Autodesk Inventor part; units mm, degrees
(part 2 of 3)
  spline S206 degree 2 poles (86.5499, 10.3817) (86.5499, 12.0564) (88.3061, 14.0423) (89.7214, 14.0423) knots 0 0 0 1 2 2 2
  spline S207 degree 2 poles (89.7214, 14.0423) (90.3587, 14.0423) (91.3442, 13.6718) (91.7073, 13.279) knots 0 0 0 1 2 2 2
  spline S208 degree 2 poles (91.7073, 13.279) (92.0778, 12.8863) (92.4705, 11.7526) (92.4705, 10.93) knots 0 0 0 1 2 2 2
  line L246 (92.4705, 10.93) -> (92.4705, 10.3002)
  line L247 (92.4705, 10.3002) -> (87.7207, 10.3002)
  spline S209 degree 2 poles (87.7207, 10.3002) (87.7207, 9.1072) (88.9211, 7.84) (89.9882, 7.84) knots 0 0 0 1 2 2 2
  spline S210 degree 2 poles (89.9882, 7.84) (90.3661, 7.84) (91.0997, 8.0105) (91.3961, 8.1439) knots 0 0 0 1 2 2 2
  spline S211 degree 2 poles (91.3961, 8.1439) (91.7073, 8.2921) (92.1371, 8.5514) (92.2779, 8.67) knots 0 0 0 1 2 2 2
  line L248 (92.2779, 8.67) -> (92.3446, 8.67)
  line L249 (92.3446, 8.67) -> (92.3446, 7.4103)
  spline S212 degree 2 poles (92.3446, 7.4103) (92.1445, 7.3288) (91.5369, 7.0916) (91.2998, 7.0249) knots 0 0 0 1 2 2 2
  spline S213 degree 2 poles (91.2998, 7.0249) (90.9663, 6.9286) (90.418, 6.8323) (90.003, 6.8323) knots 0 0 0 1 2 2 2
  spline S214 degree 2 poles (91.3442, 11.182) (91.3294, 11.6488) (91.1367, 12.3305) (90.9515, 12.5602) knots 0 0 0 1 2 2 2
  spline S215 degree 2 poles (90.9515, 12.5602) (90.7514, 12.8196) (90.1216, 13.0938) (89.6547, 13.0938) knots 0 0 0 1 2 2 2
  spline S216 degree 2 poles (89.6547, 13.0938) (89.1953, 13.0938) (88.5506, 12.8196) (88.2839, 12.5528) knots 0 0 0 1 2 2 2
  spline S217 degree 2 poles (88.2839, 12.5528) (88.0245, 12.2787) (87.7577, 11.6192) (87.7207, 11.182) knots 0 0 0 1 2 2 2
  line L250 (87.7207, 11.182) -> (91.3442, 11.182)
  line L251 (98.9173, 6.9879) -> (97.7613, 6.9879)
  line L252 (97.7613, 6.9879) -> (97.7613, 7.6844)
  spline S218 degree 2 poles (97.7613, 7.6844) (97.4946, 7.4621) (97.1018, 7.1657) (96.8351, 7.0398) knots 0 0 0 1 2 2 2
  spline S219 degree 2 poles (96.8351, 7.0398) (96.5905, 6.9212) (96.0644, 6.7952) (95.7161, 6.7952) knots 0 0 0 1 2 2 2
  spline S220 degree 2 poles (95.7161, 6.7952) (95.153, 6.7952) (94.2045, 7.2621) (93.871, 7.7141) knots 0 0 0 1 2 2 2
  spline S221 degree 2 poles (93.871, 7.7141) (93.5376, 8.1661) (93.1671, 9.4999) (93.1671, 10.3669) knots 0 0 0 1 2 2 2
  spline S222 degree 2 poles (93.1671, 10.3669) (93.1671, 11.2709) (93.6339, 12.5899) (94.0415, 13.0864) knots 0 0 0 1 2 2 2
  spline S223 degree 2 poles (94.0415, 13.0864) (94.4194, 13.531) (95.479, 14.0423) (96.0644, 14.0423) knots 0 0 0 1 2 2 2
  spline S224 degree 2 poles (96.0644, 14.0423) (96.5757, 14.0423) (97.3389, 13.8125) (97.7613, 13.5754) knots 0 0 0 1 2 2 2
  line L253 (97.7613, 13.5754) -> (97.7613, 16.5394)
  line L254 (97.7613, 16.5394) -> (98.9173, 16.5394)
  line L255 (98.9173, 16.5394) -> (98.9173, 6.9879)
  line L256 (97.7613, 8.6552) -> (97.7613, 12.6195)
  spline S225 degree 2 poles (97.7613, 12.6195) (97.3315, 12.827) (96.6498, 12.9826) (96.2571, 12.9826) knots 0 0 0 1 2 2 2
  spline S226 degree 2 poles (96.2571, 12.9826) (95.3679, 12.9826) (94.3601, 11.6488) (94.3601, 10.3891) knots 0 0 0 1 2 2 2
  spline S227 degree 2 poles (94.3601, 10.3891) (94.3601, 9.1739) (95.1307, 7.8919) (95.9829, 7.8919) knots 0 0 0 1 2 2 2
  spline S228 degree 2 poles (95.9829, 7.8919) (96.4349, 7.8919) (97.3538, 8.3069) (97.7613, 8.6552) knots 0 0 0 1 2 2 2
  line L257 (105.9272, 6.9879) -> (104.7712, 6.9879)
  line L258 (104.7712, 6.9879) -> (104.7712, 7.7437)
  spline S229 degree 2 poles (104.7712, 7.7437) (104.2377, 7.2769) (103.2818, 6.7952) (102.689, 6.7952) knots 0 0 0 1 2 2 2
  spline S230 degree 2 poles (102.689, 6.7952) (102.2444, 6.7952) (101.4515, 7.0916) (101.1625, 7.4103) knots 0 0 0 1 2 2 2
  spline S231 degree 2 poles (101.1625, 7.4103) (100.8661, 7.7289) (100.5401, 8.6996) (100.5401, 9.3962) knots 0 0 0 1 2 2 2
  line L259 (100.5401, 9.3962) -> (100.5401, 13.8496)
  line L260 (100.5401, 13.8496) -> (101.696, 13.8496)
  line L261 (101.696, 13.8496) -> (101.696, 9.9371)
  spline S232 degree 2 poles (101.696, 9.9371) (101.696, 9.3887) (101.7776, 8.67) (101.9184, 8.4032) knots 0 0 0 1 2 2 2
  spline S233 degree 2 poles (101.9184, 8.4032) (102.0591, 8.1365) (102.5408, 7.8919) (102.9928, 7.8919) knots 0 0 0 1 2 2 2
  spline S234 degree 2 poles (102.9928, 7.8919) (103.4152, 7.8919) (104.3711, 8.3736) (104.7712, 8.7218) knots 0 0 0 1 2 2 2
  line L262 (104.7712, 8.7218) -> (104.7712, 13.8496)
  line L263 (104.7712, 13.8496) -> (105.9272, 13.8496)
  line L264 (105.9272, 13.8496) -> (105.9272, 6.9879)
  line L265 (143.2657, 28.3705) -> (142.0505, 28.3705)
  line L266 (142.0505, 28.3705) -> (142.0505, 36.2474)
  line L267 (142.0505, 36.2474) -> (139.6645, 30.8899)
  line L268 (139.6645, 30.8899) -> (138.9235, 30.8899)
  line L269 (138.9235, 30.8899) -> (136.5597, 36.2474)
  line L270 (136.5597, 36.2474) -> (136.5597, 28.3705)
  line L271 (136.5597, 28.3705) -> (135.4259, 28.3705)
  line L272 (135.4259, 28.3705) -> (135.4259, 37.5145)
  line L273 (135.4259, 37.5145) -> (137.0858, 37.5145)
  line L274 (137.0858, 37.5145) -> (139.3681, 32.4238)
  line L275 (139.3681, 32.4238) -> (141.5763, 37.5145)
  line L276 (141.5763, 37.5145) -> (143.2657, 37.5145)
  line L277 (143.2657, 37.5145) -> (143.2657, 28.3705)
  spline S235 degree 2 poles (148.312, 28.1778) (147.5043, 28.1778) (146.3039, 28.6002) (145.8815, 29.0226) knots 0 0 0 1 2 2 2
  spline S236 degree 2 poles (145.8815, 29.0226) (145.3998, 29.4968) (145.0071, 30.8306) (145.0071, 31.8088) knots 0 0 0 1 2 2 2
  line L278 (145.0071, 31.8088) -> (145.0071, 37.5145)
  line L279 (145.0071, 37.5145) -> (146.2224, 37.5145)
  line L280 (146.2224, 37.5145) -> (146.2224, 31.8088)
  spline S237 degree 2 poles (146.2224, 31.8088) (146.2224, 31.1715) (146.3854, 30.3119) (146.6151, 29.9637) knots 0 0 0 1 2 2 2
  spline S238 degree 2 poles (146.6151, 29.9637) (146.8596, 29.5932) (147.7044, 29.2152) (148.312, 29.2152) knots 0 0 0 1 2 2 2
  spline S239 degree 2 poles (148.312, 29.2152) (148.8826, 29.2152) (149.7718, 29.5932) (150.0163, 29.9637) knots 0 0 0 1 2 2 2
  spline S240 degree 2 poles (150.0163, 29.9637) (150.246, 30.3119) (150.409, 31.1641) (150.409, 31.7791) knots 0 0 0 1 2 2 2
  line L281 (150.409, 31.7791) -> (150.409, 37.5145)
  line L282 (150.409, 37.5145) -> (151.6243, 37.5145)
  line L283 (151.6243, 37.5145) -> (151.6243, 31.8088)
  spline S241 degree 2 poles (151.6243, 31.8088) (151.6243, 30.8529) (151.239, 29.4894) (150.7499, 29.0226) knots 0 0 0 1 2 2 2
  spline S242 degree 2 poles (150.7499, 29.0226) (150.3127, 28.5928) (149.1567, 28.1778) (148.312, 28.1778) knots 0 0 0 1 2 2 2
  spline S243 degree 2 poles (155.9147, 28.2075) (154.9218, 28.2075) (153.5287, 28.6224) (152.9136, 28.9188) knots 0 0 0 1 2 2 2
  line L284 (152.9136, 28.9188) -> (152.9136, 30.4453)
  line L285 (152.9136, 30.4453) -> (153.0026, 30.4453)
  spline S244 degree 2 poles (153.0026, 30.4453) (153.6028, 29.8821) (155.1218, 29.2597) (155.8258, 29.2597) knots 0 0 0 1 2 2 2
  spline S245 degree 2 poles (155.8258, 29.2597) (156.8335, 29.2597) (157.8635, 30.097) (157.8635, 30.7862) knots 0 0 0 1 2 2 2
  spline S246 degree 2 poles (157.8635, 30.7862) (157.8635, 31.3345) (157.3226, 32.0162) (156.7372, 32.1867) knots 0 0 0 1 2 2 2
  spline S247 degree 2 poles (156.7372, 32.1867) (156.3148, 32.3052) (155.6109, 32.4683) (155.0848, 32.6016) knots 0 0 0 1 2 2 2
  spline S248 degree 2 poles (155.0848, 32.6016) (154.6105, 32.7276) (153.8621, 33.1055) (153.5731, 33.4093) knots 0 0 0 1 2 2 2
  spline S249 degree 2 poles (153.5731, 33.4093) (153.2915, 33.7131) (152.9803, 34.5282) (152.9803, 35.0618) knots 0 0 0 1 2 2 2
  spline S250 degree 2 poles (152.9803, 35.0618) (152.9803, 36.1733) (154.7143, 37.6775) (156.0555, 37.6775) knots 0 0 0 1 2 2 2
  spline S251 degree 2 poles (156.0555, 37.6775) (156.8261, 37.6775) (158.1896, 37.3737) (158.775, 37.0847) knots 0 0 0 1 2 2 2
  line L286 (158.775, 37.0847) -> (158.775, 35.6323)
  line L287 (158.775, 35.6323) -> (158.6861, 35.6323)
  spline S252 degree 2 poles (158.6861, 35.6323) (158.2489, 36.0325) (156.8854, 36.6253) (156.137, 36.6253) knots 0 0 0 1 2 2 2
  spline S253 degree 2 poles (156.137, 36.6253) (155.2923, 36.6253) (154.2474, 35.8324) (154.2474, 35.1877) knots 0 0 0 1 2 2 2
  spline S254 degree 2 poles (154.2474, 35.1877) (154.2474, 34.6098) (154.8625, 33.9206) (155.4405, 33.765) knots 0 0 0 1 2 2 2
  spline S255 degree 2 poles (155.4405, 33.765) (155.8258, 33.6613) (156.9447, 33.3945) (157.3152, 33.2834) knots 0 0 0 1 2 2 2
  spline S256 degree 2 poles (157.3152, 33.2834) (158.2563, 32.9944) (159.1307, 31.831) (159.1307, 30.9788) knots 0 0 0 1 2 2 2
  spline S257 degree 2 poles (159.1307, 30.9788) (159.1307, 30.4379) (158.6935, 29.4005) (158.3007, 29.0374) knots 0 0 0 1 2 2 2
  spline S258 degree 2 poles (158.3007, 29.0374) (157.8635, 28.6373) (156.752, 28.2075) (155.9147, 28.2075) knots 0 0 0 1 2 2 2
  line L288 (169.2157, 28.3705) -> (164.7549, 28.3705)
  line L289 (164.7549, 28.3705) -> (164.7549, 29.3042)
  line L290 (164.7549, 29.3042) -> (166.4147, 29.3042)
  line L291 (166.4147, 29.3042) -> (166.4147, 35.4323)
  line L292 (166.4147, 35.4323) -> (164.7549, 35.4323)
  line L293 (164.7549, 35.4323) -> (164.7549, 36.2696)
  spline S259 degree 2 poles (164.7549, 36.2696) (165.696, 36.2696) (166.5852, 36.8031) (166.6444, 37.5441) knots 0 0 0 1 2 2 2
  line L294 (166.6444, 37.5441) -> (167.5929, 37.5441)
  line L295 (167.5929, 37.5441) -> (167.5929, 29.3042)
  line L296 (167.5929, 29.3042) -> (169.2157, 29.3042)
  line L297 (169.2157, 29.3042) -> (169.2157, 28.3705)
  line L298 (170.1716, 28.3705) -> (173.2542, 37.5145)
  line L299 (173.2542, 37.5145) -> (174.751, 37.5145)
  line L300 (174.751, 37.5145) -> (177.8336, 28.3705)
  line L301 (177.8336, 28.3705) -> (176.5517, 28.3705)
  line L302 (176.5517, 28.3705) -> (175.7218, 30.927)
  line L303 (175.7218, 30.927) -> (172.2316, 30.927)
  line L304 (172.2316, 30.927) -> (171.4017, 28.3705)
  line L305 (171.4017, 28.3705) -> (170.1716, 28.3705)
  line L306 (175.3883, 31.9644) -> (173.973, 36.2696)
  line L307 (173.973, 36.2696) -> (172.5651, 31.9644)
  line L308 (172.5651, 31.9644) -> (175.3883, 31.9644)
  spline S260 degree 2 poles (121.6729, 13.1521) (120.6799, 13.1521) (119.2868, 13.5671) (118.6718, 13.8635) knots 0 0 0 1 2 2 2
  line L309 (118.6718, 13.8635) -> (118.6718, 15.39)
  line L310 (118.6718, 15.39) -> (118.7607, 15.39)
  spline S261 degree 2 poles (118.7607, 15.39) (119.3609, 14.8268) (120.88, 14.2043) (121.5839, 14.2043) knots 0 0 0 1 2 2 2
  spline S262 degree 2 poles (121.5839, 14.2043) (122.5917, 14.2043) (123.6217, 15.0417) (123.6217, 15.7308) knots 0 0 0 1 2 2 2
  spline S263 degree 2 poles (123.6217, 15.7308) (123.6217, 16.2792) (123.0808, 16.9609) (122.4954, 17.1313) knots 0 0 0 1 2 2 2
  spline S264 degree 2 poles (122.4954, 17.1313) (122.073, 17.2499) (121.3691, 17.4129) (120.8429, 17.5463) knots 0 0 0 1 2 2 2
  spline S265 degree 2 poles (120.8429, 17.5463) (120.3687, 17.6723) (119.6203, 18.0502) (119.3313, 18.354) knots 0 0 0 1 2 2 2
  spline S266 degree 2 poles (119.3313, 18.354) (119.0497, 18.6578) (118.7385, 19.4729) (118.7385, 20.0064) knots 0 0 0 1 2 2 2
  spline S267 degree 2 poles (118.7385, 20.0064) (118.7385, 21.1179) (120.4724, 22.6222) (121.8137, 22.6222) knots 0 0 0 1 2 2 2
  spline S268 degree 2 poles (121.8137, 22.6222) (122.5843, 22.6222) (123.9478, 22.3184) (124.5331, 22.0294) knots 0 0 0 1 2 2 2
  line L311 (124.5331, 22.0294) -> (124.5331, 20.577)
  line L312 (124.5331, 20.577) -> (124.4442, 20.577)
  spline S269 degree 2 poles (124.4442, 20.577) (124.007, 20.9771) (122.6436, 21.5699) (121.8952, 21.5699) knots 0 0 0 1 2 2 2
  spline S270 degree 2 poles (121.8952, 21.5699) (121.0504, 21.5699) (120.0056, 20.7771) (120.0056, 20.1324) knots 0 0 0 1 2 2 2
  spline S271 degree 2 poles (120.0056, 20.1324) (120.0056, 19.5544) (120.6206, 18.8653) (121.1986, 18.7097) knots 0 0 0 1 2 2 2
  spline S272 degree 2 poles (121.1986, 18.7097) (121.5839, 18.6059) (122.7029, 18.3392) (123.0734, 18.228) knots 0 0 0 1 2 2 2
  spline S273 degree 2 poles (123.0734, 18.228) (124.0144, 17.939) (124.8888, 16.7756) (124.8888, 15.9235) knots 0 0 0 1 2 2 2
  spline S274 degree 2 poles (124.8888, 15.9235) (124.8888, 15.3825) (124.4516, 14.3451) (124.0589, 13.982) knots 0 0 0 1 2 2 2
  spline S275 degree 2 poles (124.0589, 13.982) (123.6217, 13.5819) (122.5102, 13.1521) (121.6729, 13.1521) knots 0 0 0 1 2 2 2
  line L313 (126.1263, 13.3151) -> (126.1263, 22.4591)
  line L314 (126.1263, 22.4591) -> (131.8469, 22.4591)
  line L315 (131.8469, 22.4591) -> (131.8469, 21.3773)
  line L316 (131.8469, 21.3773) -> (127.3416, 21.3773)
  line L317 (127.3416, 21.3773) -> (127.3416, 18.8727)
  line L318 (127.3416, 18.8727) -> (131.5431, 18.8727)
  line L319 (131.5431, 18.8727) -> (131.5431, 17.7908)
  line L320 (131.5431, 17.7908) -> (127.3416, 17.7908)
  line L321 (127.3416, 17.7908) -> (127.3416, 14.397)
  line L322 (127.3416, 14.397) -> (131.8469, 14.397)
  line L323 (131.8469, 14.397) -> (131.8469, 13.3151)
  line L324 (131.8469, 13.3151) -> (126.1263, 13.3151)
  spline S276 degree 2 poles (136.7523, 13.1521) (135.8631, 13.1521) (134.3589, 13.7523) (133.8105, 14.3525) knots 0 0 0 1 2 2 2
  spline S277 degree 2 poles (133.8105, 14.3525) (133.2622, 14.9454) (132.662, 16.7238) (132.662, 17.8797) knots 0 0 0 1 2 2 2
  spline S278 degree 2 poles (132.662, 17.8797) (132.662, 19.0283) (133.2474, 20.7326) (133.8031, 21.3625) knots 0 0 0 1 2 2 2
  spline S279 degree 2 poles (133.8031, 21.3625) (134.3515, 21.9775) (135.8483, 22.6222) (136.7745, 22.6222) knots 0 0 0 1 2 2 2
  spline S280 degree 2 poles (136.7745, 22.6222) (137.234, 22.6222) (138.0417, 22.4888) (138.3825, 22.385) knots 0 0 0 1 2 2 2
  spline S281 degree 2 poles (138.3825, 22.385) (138.6789, 22.2887) (139.294, 22.0145) (139.5978, 21.8515) knots 0 0 0 1 2 2 2
  line L325 (139.5978, 21.8515) -> (139.5978, 20.3843)
  line L326 (139.5978, 20.3843) -> (139.5014, 20.3843)
  spline S282 degree 2 poles (139.5014, 20.3843) (139.3384, 20.5325) (138.8345, 20.9475) (138.4714, 21.1476) knots 0 0 0 1 2 2 2
  spline S283 degree 2 poles (138.4714, 21.1476) (138.1232, 21.3402) (137.3007, 21.5848) (136.7671, 21.5848) knots 0 0 0 1 2 2 2
  spline S284 degree 2 poles (136.7671, 21.5848) (136.1817, 21.5848) (135.1369, 21.1031) (134.7442, 20.6437) knots 0 0 0 1 2 2 2
  spline S285 degree 2 poles (134.7442, 20.6437) (134.3589, 20.1768) (133.9291, 18.7615) (133.9291, 17.8797) knots 0 0 0 1 2 2 2
  spline S286 degree 2 poles (133.9291, 17.8797) (133.9291, 16.9387) (134.3811, 15.5826) (134.7738, 15.1158) knots 0 0 0 1 2 2 2
  spline S287 degree 2 poles (134.7738, 15.1158) (135.1592, 14.6638) (136.1892, 14.2043) (136.7671, 14.2043) knots 0 0 0 1 2 2 2
  spline S288 degree 2 poles (136.7671, 14.2043) (137.2933, 14.2043) (138.1899, 14.4637) (138.5381, 14.6564) knots 0 0 0 1 2 2 2
  spline S289 degree 2 poles (138.5381, 14.6564) (138.8716, 14.849) (139.3681, 15.2492) (139.5089, 15.39) knots 0 0 0 1 2 2 2
  line L327 (139.5089, 15.39) -> (139.5978, 15.39)
  line L328 (139.5978, 15.39) -> (139.5978, 13.9376)
  spline S290 degree 2 poles (139.5978, 13.9376) (139.294, 13.7968) (138.7604, 13.5374) (138.3825, 13.4189) knots 0 0 0 1 2 2 2
  spline S291 degree 2 poles (138.3825, 13.4189) (137.9824, 13.2855) (137.3007, 13.1521) (136.7523, 13.1521) knots 0 0 0 1 2 2 2
  line L329 (142.8656, 13.3151) -> (142.8656, 21.3773)
  line L330 (142.8656, 21.3773) -> (139.7978, 21.3773)
  line L331 (139.7978, 21.3773) -> (139.7978, 22.4591)
  line L332 (139.7978, 22.4591) -> (147.1486, 22.4591)
  line L333 (147.1486, 22.4591) -> (147.1486, 21.3773)
  line L334 (147.1486, 21.3773) -> (144.0809, 21.3773)
  line L335 (144.0809, 21.3773) -> (144.0809, 13.3151)
  line L336 (144.0809, 13.3151) -> (142.8656, 13.3151)
  line L337 (151.2612, 13.3151) -> (147.7192, 13.3151)
  line L338 (147.7192, 13.3151) -> (147.7192, 14.2488)
  line L339 (147.7192, 14.2488) -> (148.8826, 14.2488)
  line L340 (148.8826, 14.2488) -> (148.8826, 21.5255)
  line L341 (148.8826, 21.5255) -> (147.7192, 21.5255)
  line L342 (147.7192, 21.5255) -> (147.7192, 22.4591)
  line L343 (147.7192, 22.4591) -> (151.2612, 22.4591)
  line L344 (151.2612, 22.4591) -> (151.2612, 21.5255)
  line L345 (151.2612, 21.5255) -> (150.0978, 21.5255)
  line L346 (150.0978, 21.5255) -> (150.0978, 14.2488)
  line L347 (150.0978, 14.2488) -> (151.2612, 14.2488)
  line L348 (151.2612, 14.2488) -> (151.2612, 13.3151)
  spline S292 degree 2 poles (159.2344, 21.4143) (159.7531, 20.8067) (160.3311, 19.0283) (160.3311, 17.8871) knots 0 0 0 1 2 2 2
  spline S293 degree 2 poles (160.3311, 17.8871) (160.3311, 16.7756) (159.7679, 14.975) (159.2344, 14.3674) knots 0 0 0 1 2 2 2
  spline S294 degree 2 poles (159.2344, 14.3674) (158.6712, 13.7301) (157.1818, 13.1225) (156.2852, 13.1225) knots 0 0 0 1 2 2 2
  spline S295 degree 2 poles (156.2852, 13.1225) (155.3589, 13.1225) (153.8769, 13.7523) (153.336, 14.3674) knots 0 0 0 1 2 2 2
  spline S296 degree 2 poles (153.336, 14.3674) (152.8099, 14.975) (152.2467, 16.7608) (152.2467, 17.8871) knots 0 0 0 1 2 2 2
  spline S297 degree 2 poles (152.2467, 17.8871) (152.2467, 19.0357) (152.8173, 20.7845) (153.3434, 21.4143) knots 0 0 0 1 2 2 2
  spline S298 degree 2 poles (153.3434, 21.4143) (153.8769, 22.0219) (155.3664, 22.6518) (156.2852, 22.6518) knots 0 0 0 1 2 2 2
  spline S299 degree 2 poles (156.2852, 22.6518) (157.2189, 22.6518) (158.7157, 21.9997) (159.2344, 21.4143) knots 0 0 0 1 2 2 2
  spline S300 degree 2 poles (159.064, 17.8871) (159.064, 18.7912) (158.6712, 20.1917) (158.3156, 20.6511) knots 0 0 0 1 2 2 2
  spline S301 degree 2 poles (158.3156, 20.6511) (157.9525, 21.1253) (156.9299, 21.5996) (156.2926, 21.5996) knots 0 0 0 1 2 2 2
  spline S302 degree 2 poles (156.2926, 21.5996) (155.6331, 21.5996) (154.6402, 21.1402) (154.2623, 20.6511) knots 0 0 0 1 2 2 2
  spline S303 degree 2 poles (154.2623, 20.6511) (153.8992, 20.1843) (153.5138, 18.7763) (153.5138, 17.8871) knots 0 0 0 1 2 2 2
  spline S304 degree 2 poles (153.5138, 17.8871) (153.5138, 16.0865) (155.0255, 14.1747) (156.2926, 14.1747) knots 0 0 0 1 2 2 2
  spline S305 degree 2 poles (156.2926, 14.1747) (157.5597, 14.1747) (159.064, 16.0865) (159.064, 17.8871) knots 0 0 0 1 2 2 2
  line L349 (168.208, 13.3151) -> (166.8445, 13.3151)
  line L350 (166.8445, 13.3151) -> (162.7986, 21.1994)
  line L351 (162.7986, 21.1994) -> (162.7986, 13.3151)
  line L352 (162.7986, 13.3151) -> (161.6649, 13.3151)
  line L353 (161.6649, 13.3151) -> (161.6649, 22.4591)
  line L354 (161.6649, 22.4591) -> (163.3914, 22.4591)
  line L355 (163.3914, 22.4591) -> (167.0742, 15.2195)
  line L356 (167.0742, 15.2195) -> (167.0742, 22.4591)
  line L357 (167.0742, 22.4591) -> (168.208, 22.4591)
  line L358 (168.208, 22.4591) -> (168.208, 13.3151)
  spline S306 degree 2 poles (180.19, 16.1236) (180.19, 15.4418) (179.6713, 14.397) (179.2415, 14.0561) knots 0 0 0 1 2 2 2
  spline S307 degree 2 poles (179.2415, 14.0561) (178.7228, 13.656) (177.5446, 13.3151) (176.611, 13.3151) knots 0 0 0 1 2 2 2
  line L359 (176.611, 13.3151) -> (173.9878, 13.3151)
  line L360 (173.9878, 13.3151) -> (173.9878, 22.4591)
  line L361 (173.9878, 22.4591) -> (176.4109, 22.4591)
  spline S308 degree 2 poles (176.4109, 22.4591) (177.389, 22.4591) (178.3671, 22.3332) (178.8118, 22.0886) knots 0 0 0 1 2 2 2
  spline S309 degree 2 poles (178.8118, 22.0886) (179.3082, 21.8293) (179.7602, 20.9771) (179.7602, 20.3991) knots 0 0 0 1 2 2 2
  spline S310 degree 2 poles (179.7602, 20.3991) (179.7602, 19.7545) (179.0785, 18.7319) (178.4783, 18.4429) knots 0 0 0 1 2 2 2
  line L362 (178.4783, 18.4429) -> (178.4783, 18.3984)
  spline S311 degree 2 poles (178.4783, 18.3984) (179.2934, 18.1761) (180.19, 16.9979) (180.19, 16.1236) knots 0 0 0 1 2 2 2
  spline S312 degree 2 poles (178.9229, 16.0717) (178.9229, 16.5904) (178.6265, 17.2573) (178.1819, 17.4944) knots 0 0 0 1 2 2 2
  spline S313 degree 2 poles (178.1819, 17.4944) (177.8929, 17.6426) (177.2112, 17.7315) (176.5813, 17.7315) knots 0 0 0 1 2 2 2
  line L363 (176.5813, 17.7315) -> (175.2031, 17.7315)
  line L364 (175.2031, 17.7315) -> (175.2031, 14.3525)
  line L365 (175.2031, 14.3525) -> (176.1886, 14.3525)
  spline S314 degree 2 poles (176.1886, 14.3525) (176.9889, 14.3525) (177.9077, 14.5008) (178.2634, 14.7379) knots 0 0 0 1 2 2 2
  spline S315 degree 2 poles (178.2634, 14.7379) (178.6043, 14.9824) (178.9229, 15.59) (178.9229, 16.0717) knots 0 0 0 1 2 2 2
  spline S316 degree 2 poles (178.4931, 20.2287) (178.4931, 20.5548) (178.2708, 21.0438) (178.0263, 21.1846) knots 0 0 0 1 2 2 2
  spline S317 degree 2 poles (178.0263, 21.1846) (177.7299, 21.3476) (177.0111, 21.4217) (176.3664, 21.4217) knots 0 0 0 1 2 2 2
  line L366 (176.3664, 21.4217) -> (175.2031, 21.4217)
  line L367 (175.2031, 21.4217) -> (175.2031, 18.7467)
  line L368 (175.2031, 18.7467) -> (176.5813, 18.7467)
  spline S318 degree 2 poles (176.5813, 18.7467) (177.1519, 18.7467) (177.6928, 18.8653) (177.9818, 19.0505) knots 0 0 0 1 2 2 2
  spline S319 degree 2 poles (177.9818, 19.0505) (178.2634, 19.2284) (178.4931, 19.7989) (178.4931, 20.2287) knots 0 0 0 1 2 2 2
  spline S320 degree 2 poles (186.8294, 17.8871) (186.8294, 15.427) (185.3993, 13.1225) (183.9099, 13.1225) knots 0 0 0 1 2 2 2
  spline S321 degree 2 poles (183.9099, 13.1225) (182.3982, 13.1225) (180.9829, 15.4715) (180.9829, 17.8797) knots 0 0 0 1 2 2 2
  spline S322 degree 2 poles (180.9829, 17.8797) (180.9829, 20.3547) (182.413, 22.6444) (183.9099, 22.6444) knots 0 0 0 1 2 2 2
  spline S323 degree 2 poles (183.9099, 22.6444) (185.4141, 22.6444) (186.8294, 20.2732) (186.8294, 17.8871) knots 0 0 0 1 2 2 2
  spline S324 degree 2 poles (185.2585, 15.101) (185.4363, 15.553) (185.5845, 16.9461) (185.5845, 17.8871) knots 0 0 0 1 2 2 2
  spline S325 degree 2 poles (185.5845, 17.8871) (185.5845, 18.8282) (185.4363, 20.2139) (185.2511, 20.6807) knots 0 0 0 1 2 2 2
  spline S326 degree 2 poles (185.2511, 20.6807) (185.0658, 21.1476) (184.4212, 21.6292) (183.9099, 21.6292) knots 0 0 0 1 2 2 2
  spline S327 degree 2 poles (183.9099, 21.6292) (183.3986, 21.6292) (182.7391, 21.1476) (182.5464, 20.6659) knots 0 0 0 1 2 2 2
  spline S328 degree 2 poles (182.5464, 20.6659) (182.3612, 20.1991) (182.2278, 18.7763) (182.2278, 17.8797) knots 0 0 0 1 2 2 2
  spline S329 degree 2 poles (182.2278, 17.8797) (182.2278, 16.9164) (182.3463, 15.6271) (182.539, 15.1232) knots 0 0 0 1 2 2 2
  spline S330 degree 2 poles (182.539, 15.1232) (182.7168, 14.649) (183.3763, 14.1377) (183.9099, 14.1377) knots 0 0 0 1 2 2 2
  spline S331 degree 2 poles (183.9099, 14.1377) (184.4137, 14.1377) (185.0732, 14.6193) (185.2585, 15.101) knots 0 0 0 1 2 2 2
  spline S332 degree 2 poles (190.4678, 21.5922) (190.1343, 21.5922) (189.4748, 21.4291) (189.1562, 21.3032) knots 0 0 0 1 2 2 2
  spline S333 degree 2 poles (189.1562, 21.3032) (188.8598, 21.1772) (188.4226, 20.9104) (188.2522, 20.7919) knots 0 0 0 1 2 2 2
  line L369 (188.2522, 20.7919) -> (188.1781, 20.7919)
  line L370 (188.1781, 20.7919) -> (188.1781, 22.0886)
  spline S334 degree 2 poles (188.1781, 22.0886) (188.5782, 22.3035) (189.9491, 22.6518) (190.5641, 22.6518) knots 0 0 0 1 2 2 2
  spline S335 degree 2 poles (190.5641, 22.6518) (191.1865, 22.6518) (192.1128, 22.3999) (192.4907, 22.1331) knots 0 0 0 1 2 2 2
  spline S336 degree 2 poles (192.4907, 22.1331) (192.8908, 21.8441) (193.3058, 21.0068) (193.3058, 20.4436) knots 0 0 0 1 2 2 2
  spline S337 degree 2 poles (193.3058, 20.4436) (193.3058, 19.6878) (192.3129, 18.5466) (191.6163, 18.3984) knots 0 0 0 1 2 2 2
  line L371 (191.6163, 18.3984) -> (191.6163, 18.3095)
  spline S338 degree 2 poles (191.6163, 18.3095) (191.9053, 18.2502) (192.5648, 17.9835) (192.8464, 17.7167) knots 0 0 0 1 2 2 2
  spline S339 degree 2 poles (192.8464, 17.7167) (193.128, 17.4574) (193.4836, 16.6274) (193.4836, 16.0272) knots 0 0 0 1 2 2 2
  spline S340 degree 2 poles (193.4836, 16.0272) (193.4836, 15.4122) (193.0613, 14.3674) (192.676, 13.9672) knots 0 0 0 1 2 2 2
  spline S341 degree 2 poles (192.676, 13.9672) (192.2758, 13.5523) (191.1421, 13.1225) (190.4233, 13.1225) knots 0 0 0 1 2 2 2
  spline S342 degree 2 poles (190.4233, 13.1225) (189.7342, 13.1225) (188.3855, 13.4559) (187.9261, 13.6856) knots 0 0 0 1 2 2 2
  line L372 (187.9261, 13.6856) -> (187.9261, 14.9824)
  line L373 (187.9261, 14.9824) -> (188.015, 14.9824)
  spline S343 degree 2 poles (188.015, 14.9824) (188.4004, 14.7008) (189.7045, 14.1821) (190.3492, 14.1821) knots 0 0 0 1 2 2 2
  spline S344 degree 2 poles (190.3492, 14.1821) (190.7271, 14.1821) (191.4829, 14.4192) (191.7349, 14.6934) knots 0 0 0 1 2 2 2
  spline S345 degree 2 poles (191.7349, 14.6934) (191.9794, 14.9676) (192.2388, 15.6197) (192.2388, 16.1161) knots 0 0 0 1 2 2 2
  spline S346 degree 2 poles (192.2388, 16.1161) (192.2388, 16.6126) (191.9498, 17.2573) (191.6904, 17.4425) knots 0 0 0 1 2 2 2
  spline S347 degree 2 poles (191.6904, 17.4425) (191.4311, 17.6278) (190.7271, 17.7686) (190.3121, 17.7686) knots 0 0 0 1 2 2 2
  line L374 (190.3121, 17.7686) -> (189.7934, 17.7686)
  line L375 (189.7934, 17.7686) -> (189.7934, 18.7838)
  line L376 (189.7934, 18.7838) -> (190.201, 18.7838)
  spline S348 degree 2 poles (190.201, 18.7838) (191.0235, 18.7838) (192.0609, 19.5692) (192.0609, 20.3176) knots 0 0 0 1 2 2 2
  spline S349 degree 2 poles (192.0609, 20.3176) (192.0609, 20.6659) (191.7942, 21.1624) (191.5793, 21.3106) knots 0 0 0 1 2 2 2
  spline S350 degree 2 poles (191.5793, 21.3106) (191.3496, 21.4662) (190.7864, 21.5922) (190.4678, 21.5922) knots 0 0 0 1 2 2 2
  dimension "d10" = 203.2
  dimension "d11" = 50.8
  dimension "d12" = 80.6634
  dimension "d13" = 24.7194
  dimension "d14" = 102.5205
  dimension "d15" = 45.5358
  dimension "d16" = 2.6321
  dimension "d17" = 13.0403
  dimension "d18" = 6.672
  dimension "d19" = 6.672
  constraints: 4 other
  measures "d10" distance of L0.end L1.end
  measures "d11" distance of L1.end L2.end
  measures "d12" distance of L8.start L8.end
  measures "d13" distance of L10.end L8.start
  measures "d14" distance of L4.start L4.end
  measures "d15" distance of L6.end L4.start
  measures "d16" distance between parallel lines of L1 L4
  measures "d17" distance between parallel lines of L1 L8
  measures "d18" distance between parallel lines of L2 L7
  measures "d19" distance between parallel lines of L5 L11
extrude "Extrusion3" cut sketch "Sketch3" against normal blind 5.08 contours S0 S1 L12 L13 S2 S3 S4 L14 L15 L16 L17 L18 | S5 S6 L19 L20 L21 S7 S8 S9 S10 L22 L23 L24 S11 S12 | S13 L25 L26 S14 S15 S16 S17 S18 S19 S20 S21 L27 L28 S22 S23 S24 S25 S26 S27 S28 | L29 L30 L31 L32 L33 L34 L35 L36 | L37 L38 L39 L40 L41 L42 L43 L44 L45 L46 L47 L48 | L49 L50 L51 L52 L53 L54 L55 L56 L57 L58 | L59 L60 L61 L62 L63 L64 L65 L66 | L70 L71 L72 L73 L74 L75 | L76 L77 L78 L79 L80 L81 | L82 L83 L84 L85 L86 L87 L88 L89 L90 L91 L92 L93 | L94 L95 L96 L97 L98 L99 L100 L101 L102 L103 | L104 L105 L106 L107 L108 L109 L110 L111 | L115 L116 L117 L118 L119 L120 S29 L121 L122 L123 L124 | L125 L126 L127 L128 L129 L130 L131 L132 L133 L134 L135 | S30 S31 S32 L139 L140 S33 S34 S35 S36 S37 S38 S39 L141 L142 L143 L144 L145 S40 S41 S42 | S43 S44 S45 S46 S47 S48 S49 L146 L147 S50 S51 S52 S53 S54 | S62 S63 S64 S65 S66 S67 S68 L148 L149 S69 S70 S71 S72 S73 | S81 S82 S83 S84 | L150 L151 L152 L153 L154 L155 L156 | L157 L158 L159 L160 L161 L162 S93 L163 L164 L165 L166 | S94 S95 L167 L168 S96 S97 S98 L169 L170 L171 L172 L173 | L174 L175 L176 L177 | S99 S100 L178 L179 L180 L181 L182 S101 S102 | S107 S108 S109 S110 S111 S112 L184 S113 S114 S115 L185 L186 S116 S117 S118 L187 L188 L189 | L191 L192 L193 L194 | L195 L196 L197 L198 | S123 S124 S125 S126 L199 L200 S127 S128 S129 L201 L202 S130 S131 | L204 L205 S136 S137 S138 L206 L207 L208 L209 L210 S139 S140 L211 | S141 L212 L213 S142 S143 S144 S145 L214 L215 L216 L217 S146 S147 S148 S149 S150 L218 S151 S152 S153 S154 | L220 L221 S159 S160 S161 L222 L223 L224 S162 S163 S164 L225 L226 L227 | S165 S166 S167 S168 S169 L228 L229 S170 S171 S172 S173 S174 L230 L231 S175 S176 | S177 L232 L233 S178 S179 S180 S181 S182 S183 S184 S185 S186 L234 L235 S187 S188 S189 S190 S191 S192 S193 | L236 L237 S194 S195 S196 S197 S198 S199 S200 L238 L239 L240 | L242 L243 L244 L245 | S205 S206 S207 S208 L246 L247 S209 S210 S211 L248 L249 S212 S213 | L251 L252 S218 S219 S220 S221 S222 S223 S224 L253 L254 L255 | L257 L258 S229 S230 S231 L259 L260 L261 S232 S233 S234 L262 L263 L264 | L265 L266 L267 L268 L269 L270 L271 L272 L273 L274 L275 L276 L277 | S235 S236 L278 L279 L280 S237 S238 S239 S240 L281 L282 L283 S241 S242 | S243 L284 L285 S244 S245 S246 S247 S248 S249 S250 S251 L286 L287 S252 S253 S254 S255 S256 S257 S258 | L288 L289 L290 L291 L292 L293 S259 L294 L295 L296 L297 | L298 L299 L300 L301 L302 L303 L304 L305 | S260 L309 L310 S261 S262 S263 S264 S265 S266 S267 S268 L311 L312 S269 S270 S271 S272 S273 S274 S275 | L313 L314 L315 L316 L317 L318 L319 L320 L321 L322 L323 L324 | S276 S277 S278 S279 S280 S281 L325 L326 S282 S283 S284 S285 S286 S287 S288 S289 L327 L328 S290 S291 | L329 L330 L331 L332 L333 L334 L335 L336 | L337 L338 L339 L340 L341 L342 L343 L344 L345 L346 L347 L348 | S292 S293 S294 S295 S296 S297 S298 S299 | L349 L350 L351 L352 L353 L354 L355 L356 L357 L358 | S306 S307 L359 L360 L361 S308 S309 S310 L362 S311 | S320 S321 S322 S323 | S332 S333 L369 L370 S334 S335 S336 S337 L371 S338 S339 S340 S341 S342 L372 L373 S343 S344 S345 S346 S347 L374 L375 L376 S348 S349 S350
sketch "Sketch4" plane through (203.2, 0, 50.8) normal (1, 0, 0) x (0, 0, -1)
  line L0 (0, 0) -> (50.8, 0) projected
  line L1 (0, 0) -> (0, -25.4) projected
  line L2 (50.8, -25.4) -> (0, -25.4) projected
  line L3 (50.8, 0) -> (50.8, -25.4) projected
  line L4 (6.1053, -3.5259) -> (44.6947, -3.5259) construction
  line L5 (44.6947, -3.5259) -> (44.6947, -21.8741) construction
  line L6 (44.6947, -21.8741) -> (6.1053, -21.8741) construction
  line L7 (6.1053, -21.8741) -> (6.1053, -3.5259) construction
  spline S0 degree 2 poles (9.9315, -17.4424) (8.9608, -17.4424) (7.3528, -16.8496) (6.7748, -16.2494) knots 0 0 0 1 2 2 2
  spline S1 degree 2 poles (6.7748, -16.2494) (6.1969, -15.6418) (5.5818, -13.8486) (5.5818, -12.6852) knots 0 0 0 1 2 2 2
  spline S2 degree 2 poles (5.5818, -12.6852) (5.5818, -11.5811) (6.2043, -9.8323) (6.7823, -9.2099) knots 0 0 0 1 2 2 2
  spline S3 degree 2 poles (6.7823, -9.2099) (7.338, -8.6097) (8.9682, -7.9576) (9.9389, -7.9576) knots 0 0 0 1 2 2 2
  spline S4 degree 2 poles (9.9389, -7.9576) (10.4058, -7.9576) (11.2505, -8.0909) (11.6358, -8.2095) knots 0 0 0 1 2 2 2
  spline S5 degree 2 poles (11.6358, -8.2095) (11.9471, -8.2984) (12.7029, -8.6245) (12.9326, -8.743) knots 0 0 0 1 2 2 2
  line L8 (12.9326, -8.743) -> (12.9326, -10.2102)
  line L9 (12.9326, -10.2102) -> (12.8289, -10.2102)
  spline S6 degree 2 poles (12.8289, -10.2102) (12.5991, -10.0102) (12.1175, -9.6471) (11.6729, -9.4396) knots 0 0 0 1 2 2 2
  spline S7 degree 2 poles (11.6729, -9.4396) (11.3024, -9.2543) (10.3465, -9.0098) (9.7981, -9.0098) knots 0 0 0 1 2 2 2
  spline S8 degree 2 poles (9.7981, -9.0098) (8.4792, -9.0098) (6.8489, -10.9957) (6.8489, -12.6481) knots 0 0 0 1 2 2 2
  spline S9 degree 2 poles (6.8489, -12.6481) (6.8489, -13.567) (7.2787, -14.9452) (7.6863, -15.4195) knots 0 0 0 1 2 2 2
  spline S10 degree 2 poles (7.6863, -15.4195) (8.079, -15.8937) (9.1905, -16.3902) (9.8871, -16.3902) knots 0 0 0 1 2 2 2
  spline S11 degree 2 poles (9.8871, -16.3902) (10.3984, -16.3902) (11.4209, -16.242) (11.7692, -16.0938) knots 0 0 0 1 2 2 2
  line L10 (11.7692, -16.0938) -> (11.7692, -13.73)
  line L11 (11.7692, -13.73) -> (9.6499, -13.73)
  line L12 (9.6499, -13.73) -> (9.6499, -12.6629)
  line L13 (9.6499, -12.6629) -> (12.9696, -12.6629)
  line L14 (12.9696, -12.6629) -> (12.9696, -16.657)
  spline S12 degree 2 poles (12.9696, -16.657) (12.7399, -16.7607) (11.9545, -17.0793) (11.621, -17.1757) knots 0 0 0 1 2 2 2
  spline S13 degree 2 poles (11.621, -17.1757) (11.169, -17.3091) (10.4428, -17.4424) (9.9315, -17.4424) knots 0 0 0 1 2 2 2
  line L15 (14.4961, -17.2646) -> (14.4961, -8.1206)
  line L16 (14.4961, -8.1206) -> (20.2167, -8.1206)
  line L17 (20.2167, -8.1206) -> (20.2167, -9.2025)
  line L18 (20.2167, -9.2025) -> (15.7114, -9.2025)
  line L19 (15.7114, -9.2025) -> (15.7114, -11.7071)
  line L20 (15.7114, -11.7071) -> (19.9129, -11.7071)
  line L21 (19.9129, -11.7071) -> (19.9129, -12.7889)
  line L22 (19.9129, -12.7889) -> (15.7114, -12.7889)
  line L23 (15.7114, -12.7889) -> (15.7114, -16.1827)
  line L24 (15.7114, -16.1827) -> (20.2167, -16.1827)
  line L25 (20.2167, -16.1827) -> (20.2167, -17.2646)
  line L26 (20.2167, -17.2646) -> (14.4961, -17.2646)
  line L27 (24.7368, -17.2646) -> (21.1948, -17.2646)
  line L28 (21.1948, -17.2646) -> (21.1948, -16.3309)
  line L29 (21.1948, -16.3309) -> (22.3582, -16.3309)
  line L30 (22.3582, -16.3309) -> (22.3582, -9.0543)
  line L31 (22.3582, -9.0543) -> (21.1948, -9.0543)
  line L32 (21.1948, -9.0543) -> (21.1948, -8.1206)
  line L33 (21.1948, -8.1206) -> (24.7368, -8.1206)
  line L34 (24.7368, -8.1206) -> (24.7368, -9.0543)
  line L35 (24.7368, -9.0543) -> (23.5734, -9.0543)
  line L36 (23.5734, -9.0543) -> (23.5734, -16.3309)
  line L37 (23.5734, -16.3309) -> (24.7368, -16.3309)
  line L38 (24.7368, -16.3309) -> (24.7368, -17.2646)
  spline S14 degree 2 poles (28.7901, -17.4276) (27.7972, -17.4276) (26.4041, -17.0126) (25.789, -16.7162) knots 0 0 0 1 2 2 2
  line L39 (25.789, -16.7162) -> (25.789, -15.1898)
  line L40 (25.789, -15.1898) -> (25.8779, -15.1898)
  spline S15 degree 2 poles (25.8779, -15.1898) (26.4782, -15.7529) (27.9972, -16.3754) (28.7012, -16.3754) knots 0 0 0 1 2 2 2
  spline S16 degree 2 poles (28.7012, -16.3754) (29.7089, -16.3754) (30.7389, -15.538) (30.7389, -14.8489) knots 0 0 0 1 2 2 2
  spline S17 degree 2 poles (30.7389, -14.8489) (30.7389, -14.3006) (30.198, -13.6188) (29.6126, -13.4484) knots 0 0 0 1 2 2 2
  spline S18 degree 2 poles (29.6126, -13.4484) (29.1902, -13.3299) (28.4863, -13.1668) (27.9602, -13.0335) knots 0 0 0 1 2 2 2
  spline S19 degree 2 poles (27.9602, -13.0335) (27.4859, -12.9075) (26.7375, -12.5296) (26.4485, -12.2258) knots 0 0 0 1 2 2 2
  spline S20 degree 2 poles (26.4485, -12.2258) (26.1669, -11.9219) (25.8557, -11.1068) (25.8557, -10.5733) knots 0 0 0 1 2 2 2
  spline S21 degree 2 poles (25.8557, -10.5733) (25.8557, -9.4618) (27.5897, -7.9576) (28.9309, -7.9576) knots 0 0 0 1 2 2 2
  spline S22 degree 2 poles (28.9309, -7.9576) (29.7015, -7.9576) (31.065, -8.2614) (31.6504, -8.5504) knots 0 0 0 1 2 2 2
  line L41 (31.6504, -8.5504) -> (31.6504, -10.0027)
  line L42 (31.6504, -10.0027) -> (31.5615, -10.0027)
  spline S23 degree 2 poles (31.5615, -10.0027) (31.1243, -9.6026) (29.7608, -9.0098) (29.0124, -9.0098) knots 0 0 0 1 2 2 2
  spline S24 degree 2 poles (29.0124, -9.0098) (28.1677, -9.0098) (27.1228, -9.8027) (27.1228, -10.4473) knots 0 0 0 1 2 2 2
  spline S25 degree 2 poles (27.1228, -10.4473) (27.1228, -11.0253) (27.7379, -11.7145) (28.3159, -11.8701) knots 0 0 0 1 2 2 2
  spline S26 degree 2 poles (28.3159, -11.8701) (28.7012, -11.9738) (29.8201, -12.2406) (30.1906, -12.3517) knots 0 0 0 1 2 2 2
  spline S27 degree 2 poles (30.1906, -12.3517) (31.1317, -12.6407) (32.0061, -13.8041) (32.0061, -14.6563) knots 0 0 0 1 2 2 2
  spline S28 degree 2 poles (32.0061, -14.6563) (32.0061, -15.1972) (31.5689, -16.2346) (31.1761, -16.5977) knots 0 0 0 1 2 2 2
  spline S29 degree 2 poles (31.1761, -16.5977) (30.7389, -16.9978) (29.6274, -17.4276) (28.7901, -17.4276) knots 0 0 0 1 2 2 2
  line L43 (33.2435, -17.2646) -> (33.2435, -8.1206)
  line L44 (33.2435, -8.1206) -> (38.9641, -8.1206)
  line L45 (38.9641, -8.1206) -> (38.9641, -9.2025)
  line L46 (38.9641, -9.2025) -> (34.4588, -9.2025)
  line L47 (34.4588, -9.2025) -> (34.4588, -11.7071)
  line L48 (34.4588, -11.7071) -> (38.6603, -11.7071)
  line L49 (38.6603, -11.7071) -> (38.6603, -12.7889)
  line L50 (38.6603, -12.7889) -> (34.4588, -12.7889)
  line L51 (34.4588, -12.7889) -> (34.4588, -16.1827)
  line L52 (34.4588, -16.1827) -> (38.9641, -16.1827)
  line L53 (38.9641, -16.1827) -> (38.9641, -17.2646)
  line L54 (38.9641, -17.2646) -> (33.2435, -17.2646)
  line L55 (45.5961, -17.2646) -> (40.2979, -17.2646)
  line L56 (40.2979, -17.2646) -> (40.2979, -8.1206)
  line L57 (40.2979, -8.1206) -> (41.5131, -8.1206)
  line L58 (41.5131, -8.1206) -> (41.5131, -16.1827)
  line L59 (41.5131, -16.1827) -> (45.5961, -16.1827)
  line L60 (45.5961, -16.1827) -> (45.5961, -17.2646)
  dimension "d22" = 50.8
  dimension "d23" = 25.4
  dimension "d24" = 38.5894
  dimension "d25" = 18.3482
  dimension "d26" = 6.1053
  dimension "d27" = 3.5259
  constraints: 2 other
  measures "d22" distance of L0.start L0.end
  measures "d23" distance of L0.start L1.end
  measures "d24" distance of L4.start L4.end
  measures "d25" distance of L6.end L4.start
  measures "d26" distance between parallel lines of L1 L7
  measures "d27" distance between parallel lines of L0 L4
extrude "Extrusion4" cut sketch "Sketch4" against normal blind 5.08 contours S0 S1 S2 S3 S4 S5 L8 L9 S6 S7 S8 S9 S10 S11 L10 L11 L12 L13 L14 S12 S13 | L15 L16 L17 L18 L19 L20 L21 L22 L23 L24 L25 L26 | L27 L28 L29 L30 L31 L32 L33 L34 L35 L36 L37 L38 | S14 L39 L40 S15 S16 S17 S18 S19 S20 S21 S22 L41 L42 S23 S24 S25 S26 S27 S28 S29 | L43 L44 L45 L46 L47 L48 L49 L50 L51 L52 L53 L54 | L55 L56 L57 L58 L59 L60